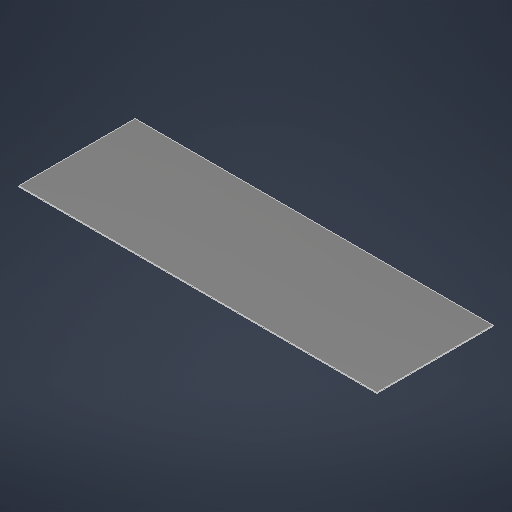
# Autodesk Inventor part: Floor, Uncutt
Saved by Autodesk Inventor 2026 (Build 300175000, 175)
## iProperties
Created: 2025-10-27
Part Number: Floor, Uncutt
Material: Acetal Resin, Black
Document SubType Name: Modeling
Designer: Brandon Portillo
Density: 1.425 g/cm^3
Appearance: Smooth - Black
Author: Brandon Portillo
Autodesk Inventor part; units mm, degrees
ref_plane "YZ Plane" through (0, 0, 0) normal (1, 0, 0) x (0, 1, 0)
ref_plane "XZ Plane" through (0, 0, 0) normal (0, 1, 0) x (-1, 0, 0)
ref_plane "XY Plane" through (0, 0, 0) normal (0, 0, 1) x (1, 0, 0)
sketch "Sketch1" plane through (0, 0, 0) normal (0, 1, 0) x (-1, 0, 0)
  line L0 (0, 0) -> (-10000, 0)
  line L1 (-10000, 0) -> (-10000, -3250)
  line L2 (-10000, -3250) -> (0, -3250)
  line L3 (0, -3250) -> (0, 0)
  dimension "d0" = 10000
  dimension "d1" = 3250
  constraints: 8 end point, 2 parallel, 1 horizontal, 1 perpendicular
  measures "d0" distance of L2.end L1.end
  measures "d1" distance of L1.end L0.end
extrude "Extrusion1" add sketch "Sketch1" along normal blind 25
body "Solid1"
